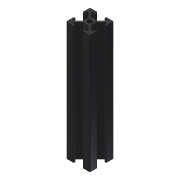
# Autodesk Inventor part: 8020-2519
Saved by Autodesk Inventor 2014 (Build 180170000, 170)
## iProperties
Created: 2014-08-06
Part Number: 8020-2519
Material: Generic
Document SubType Name: Modeling
Designer: Peele
Density: 1 g/cm^3
Appearance: Dark Gray
Author: Peele
Autodesk Inventor part; units mm, degrees
ref_plane "YZ Plane" through (0, 0, 0) normal (1, 0, 0) x (0, 1, 0)
ref_plane "XZ Plane" through (0, 0, 0) normal (0, 1, 0) x (-1, 0, 0)
ref_plane "XY Plane" through (0, 0, 0) normal (0, 0, 1) x (1, 0, 0)
sketch "Sketch1" plane through (0, 0, 0) normal (0, 0, 1) x (1, 0, 0)
  line L0 (-4.38, -4.38) -> (4.38, -4.38)
  line L1 (4.38, -4.38) -> (4.38, 4.38)
  line L2 (4.38, 4.38) -> (-4.38, 4.38)
  line L3 (-4.38, 4.38) -> (-4.38, -4.38)
  line L4 (-4.38, -4.38) -> (4.38, 4.38) construction
  line L5 (4.38, -4.38) -> (-4.38, 4.38) construction
  circle A0 centre (0, 0) radius 2.5
  dimension "d0" = 8.76
  dimension "d1" = 5
  constraints: 12 end point, 2 midpoint, 2 parallel, 2 perpendicular, 1 centre point, 1 coincident, 1 horizontal
  measures "d0" distance of L1.end L2.end
  measures "d1" diameter of A0
extrude "Extrusion1" add sketch "Sketch1" along normal mid plane 125
sketch "Sketch2" plane through (0, 0, 0) normal (0, 0, 1) x (1, 0, 0)
  line L0 (-4.38, 2.8668) -> (-10.36, 8.8468)
  line L1 (-10.36, 8.8468) -> (-10.36, 4.4)
  line L2 (-10.36, 4.4) -> (-12.5, 4.4)
  line L3 (-12.5, 4.4) -> (-12.5, 12.5)
  line L4 (-12.5, 12.5) -> (-4.4, 12.5)
  line L5 (-4.4, 12.5) -> (-4.4, 10.36)
  line L6 (-4.4, 10.36) -> (-8.8468, 10.36)
  line L7 (-8.8468, 10.36) -> (-2.8668, 4.38)
  line L8 (-2.8668, 4.38) -> (-4.38, 2.8668)
  line L9 (-4.38, 4.38) -> (4.38, 4.38) projected
  line L10 (-4.38, -4.38) -> (-4.38, 4.38) projected
  point P0 (0, 0)
  dimension "d4" = 12.5
  dimension "d5" = 2.14
  dimension "d6" = 8.1
  dimension "d7" = 2.14
  constraints: 18 end point, 6 perpendicular, 4 equal length, 2 point on line, 1 parallel, 1 vertical
  measures "d4" distance from line of point (0, 0) L4
  measures "d5" distance between parallel lines of L4 L6
  measures "d6" distance of L3.end L4.end
  measures "d7" distance between parallel lines of L0 L7
extrude "Extrusion2" add sketch "Sketch2" along normal up to surface (125 mm away) from surface at -62.5 contours L0 L1 L2 L3 L4 L5 L6 L7 L9 L10
pattern_circular "Circular Pattern1" count 4 over 360 about axis through (0, 0, 0) along (0, 0, 1) of "Extrusion2"
fillet "Fillet9" radius 1 20 edges at (12.5, 4.4, 0) (10.36, 4.4, 0) (12.5, 12.5, 0) (4.4, 10.36, 0) (4.4, 12.5, 0) (-4.4, 12.5, 0) (-12.5, 12.5, 0) (-12.5, 4.4, 0) (-4.4, 10.36, 0) (-10.36, 4.4, 0) (-10.36, -4.4, 0) (-4.4, -10.36, 0) (-4.4, -12.5, 0) (12.5, -12.5, 0) (4.4, -12.5, 0) (12.5, -4.4, 0) (10.36, -4.4, 0) (4.4, -10.36, 0) (-12.5, -4.4, 0) (-12.5, -12.5, 0)
fillet "Fillet10" radius 0.75 16 edges at (8.8468, 10.36, 0) (10.36, 8.8468, 0) (-8.8468, 10.36, 0) (-10.36, 8.8468, 0) (-8.8468, -10.36, 0) (-10.36, -8.8468, 0) (10.36, -8.8468, 0) (8.8468, -10.36, 0) (-4.38, 2.8668, 0) (-4.38, -2.8668, 0) (4.38, -2.8668, 0) (4.38, 2.8668, 0) (-2.8668, -4.38, 0) (2.8668, -4.38, 0) (-2.8668, 4.38, 0) (2.8668, 4.38, 0)
fillet "Fillet11" radius 0.75 146 edges at (-2.8431, 4.4371, 62.5) (-5.3265, 6.8397, 62.5) (-7.729, 9.897, 62.5) (-6.2181, 10.36, 62.5) (-4.6929, 10.6529, 62.5) (-4.4, 11.43, 62.5) (-4.6929, 12.2071, 62.5) (-8.45, 12.5, 62.5) (-12.2071, 12.2071, 62.5) (-12.5, 8.45, 62.5) (-12.2071, 4.6929, 62.5) (-11.43, 4.4, 62.5) (-10.6529, 4.6929, 62.5) (-10.36, 6.2181, 62.5) (-9.897, 7.729, 62.5) (-6.8397, 5.3265, 62.5) (-4.4371, 2.8431, 62.5) (-4.38, 0, 62.5) (-4.4371, -2.8431, 62.5) (-6.8397, -5.3265, 62.5) (-9.897, -7.729, 62.5) (-10.36, -6.2181, 62.5) (-10.6529, -4.6929, 62.5) (-11.43, -4.4, 62.5) (-12.2071, -4.6929, 62.5) (-12.5, -8.45, 62.5) (-12.2071, -12.2071, 62.5) (-8.45, -12.5, 62.5) (-4.6929, -12.2071, 62.5) (-4.4, -11.43, 62.5) (-4.6929, -10.6529, 62.5) (-6.2181, -10.36, 62.5) (-7.729, -9.897, 62.5) (-5.3265, -6.8397, 62.5) (-2.8431, -4.4371, 62.5) (0, -4.38, 62.5) (2.8431, -4.4371, 62.5) (5.3265, -6.8397, 62.5) (7.729, -9.897, 62.5) (6.2181, -10.36, 62.5) (4.6929, -10.6529, 62.5) (4.4, -11.43, 62.5) (4.6929, -12.2071, 62.5) (8.45, -12.5, 62.5) (12.2071, -12.2071, 62.5) (12.5, -8.45, 62.5) (12.2071, -4.6929, 62.5) (11.43, -4.4, 62.5) (10.6529, -4.6929, 62.5) (10.36, -6.2181, 62.5) (9.897, -7.729, 62.5) (6.8397, -5.3265, 62.5) (4.4371, -2.8431, 62.5) (4.38, 0, 62.5) (4.4371, 2.8431, 62.5) (6.8397, 5.3265, 62.5) (9.897, 7.729, 62.5) (10.36, 6.2181, 62.5) (10.6529, 4.6929, 62.5) (11.43, 4.4, 62.5) (12.2071, 4.6929, 62.5) (12.5, 8.45, 62.5) (12.2071, 12.2071, 62.5) (8.45, 12.5, 62.5) (4.6929, 12.2071, 62.5) (4.4, 11.43, 62.5) (4.6929, 10.6529, 62.5) (6.2181, 10.36, 62.5) (7.729, 9.897, 62.5) (5.3265, 6.8397, 62.5) (2.8431, 4.4371, 62.5) (0, 4.38, 62.5) (-2.5, 0, 62.5) (-9.897, 7.729, -62.5) (-10.36, 6.2181, -62.5) (-10.6529, 4.6929, -62.5) (-11.43, 4.4, -62.5) (-12.2071, 4.6929, -62.5) (-12.5, 8.45, -62.5) (-12.2071, 12.2071, -62.5) (-8.45, 12.5, -62.5) (-4.6929, 12.2071, -62.5) (-4.4, 11.43, -62.5) (-4.6929, 10.6529, -62.5) (-6.2181, 10.36, -62.5) (-7.729, 9.897, -62.5) (-5.3265, 6.8397, -62.5) (-2.8431, 4.4371, -62.5) (0, 4.38, -62.5) (2.8431, 4.4371, -62.5) (5.3265, 6.8397, -62.5) (7.729, 9.897, -62.5) (6.2181, 10.36, -62.5) (4.6929, 10.6529, -62.5) (4.4, 11.43, -62.5) (4.6929, 12.2071, -62.5) (8.45, 12.5, -62.5) (12.2071, 12.2071, -62.5) (12.5, 8.45, -62.5) (12.2071, 4.6929, -62.5) (11.43, 4.4, -62.5) (10.6529, 4.6929, -62.5) (10.36, 6.2181, -62.5) (9.897, 7.729, -62.5) (6.8397, 5.3265, -62.5) (4.4371, 2.8431, -62.5) (4.38, 0, -62.5) (4.4371, -2.8431, -62.5) (6.8397, -5.3265, -62.5) (9.897, -7.729, -62.5) (10.36, -6.2181, -62.5) (10.6529, -4.6929, -62.5) (11.43, -4.4, -62.5) (12.2071, -4.6929, -62.5) (12.5, -8.45, -62.5) (12.2071, -12.2071, -62.5) (8.45, -12.5, -62.5) (4.6929, -12.2071, -62.5) (4.4, -11.43, -62.5) (4.6929, -10.6529, -62.5) (6.2181, -10.36, -62.5) (7.729, -9.897, -62.5) (5.3265, -6.8397, -62.5) (2.8431, -4.4371, -62.5) (0, -4.38, -62.5) (-2.8431, -4.4371, -62.5) (-5.3265, -6.8397, -62.5) (-7.729, -9.897, -62.5) (-6.2181, -10.36, -62.5) (-4.6929, -10.6529, -62.5) (-4.4, -11.43, -62.5) (-4.6929, -12.2071, -62.5) (-8.45, -12.5, -62.5) (-12.2071, -12.2071, -62.5) (-12.5, -8.45, -62.5) (-12.2071, -4.6929, -62.5) (-11.43, -4.4, -62.5) (-10.6529, -4.6929, -62.5) (-10.36, -6.2181, -62.5) (-9.897, -7.729, -62.5) (-6.8397, -5.3265, -62.5) (-4.4371, -2.8431, -62.5) (-4.38, 0, -62.5) (-4.4371, 2.8431, -62.5) (-6.8397, 5.3265, -62.5) (-2.5, 0, -62.5)
equation "\"d7\" = d5"
body "Solid1"
